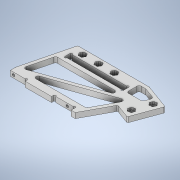
# Autodesk Inventor part: Trunk_vertical_frame_01
Saved by Autodesk Inventor 2020.4 (Build 244396000, 396)
## iProperties
Created: 2021-09-11
Part Number: Trunk_vertical_frame_01
Material: アルミニウム 2014-T4
Document SubType Name: Modeling
Designer: Masato Kubotera
Density: 2.8 g/cm^3
Appearance: 滑らか - 淡い灰色
Mass: 32.437 g
Surface Area: 89.3164 cm^2
Volume: 11.5847 cm^3
Author: Masato Kubotera
Autodesk Inventor part; units mm, degrees
ref_plane "YZ Plane" through (0, 0, 0) normal (1, 0, 0) x (0, 1, 0)
ref_plane "XZ Plane" through (0, 0, 0) normal (0, 1, 0) x (-1, 0, 0)
ref_plane "XY Plane" through (0, 0, 0) normal (0, 0, 1) x (1, 0, 0)
derived "Trunk_vertical_frame_03.ipt"
sketch "スケッチ1" plane through (0, 0, 0) normal (0, 0, 1) x (1, 0, 0)
  circle A0 centre (0, 0) radius 11 projected
  line L0 (1, 13.5) -> (28, 13.5) construction
  line L1 (28, 13.5) -> (28, -13.5) construction
  line L2 (28, -13.5) -> (1, -13.5) construction
  line L3 (1, -13.5) -> (1, 13.5) construction
  line L4 (1, 13.5) -> (28, -13.5) construction
  line L5 (28, 13.5) -> (1, -13.5) construction
  line L6 (-12, 16) -> (39.5, 16) construction
  line L7 (39.5, 16) -> (39.5, -16) construction
  line L8 (39.5, -16) -> (-12, -16) construction
  line L9 (-12, -16) -> (-12, 16) construction
  line L10 (-12, 16) -> (39.5, -16) construction
  line L11 (39.5, 16) -> (-12, -16) construction
  circle A1 centre (1, 13.5) radius 1.35 projected
  arc A2 (0, 16) -> (-12, 10.583) centre (0, 0) ccw construction
  line L12 (-12, 0) -> (39.5, 0) projected
  circle A3 centre (28, 13.5) radius 1.35 projected
  arc A4 (-12, -10.583) -> (0, -16) centre (0, 0) ccw construction
  circle A5 centre (28, -13.5) radius 1.35 projected
  circle A6 centre (1, -13.5) radius 1.35 projected
  arc A7 (0, 16.01) -> (-12.01, 10.5868) centre (0, 0) ccw projected
  line L13 (0, 16.01) -> (39.51, 16.01) projected
  line L14 (39.51, 16.01) -> (39.51, 13.26) projected
  line L15 (-12.01, 10.5868) -> (-12.01, 0) projected
  arc A8 (-11.4729, 11.1666) -> (-12.01, 9.8444) centre (-11.0278, 10.2156) ccw projected
  line L16 (-12.01, 10.5868) -> (-11.0278, 10.2156) construction
  arc A9 (39.51, 14.5251) -> (38.0251, 16.01) centre (38.7675, 15.2675) ccw projected
  line L17 (38.7675, 15.2675) -> (39.51, 16.01) construction
  arc A10 (38.0251, -16.01) -> (39.51, -14.5251) centre (38.7675, -15.2675) ccw projected
  line L18 (-12.01, -10.5868) -> (-12.01, 0) projected
  arc A11 (-12.01, -9.8444) -> (-11.4729, -11.1666) centre (-11.0278, -10.2156) ccw projected
  arc A12 (-12.01, -10.5868) -> (0, -16.01) centre (0, 0) ccw projected
  line L19 (0, -16.01) -> (39.51, -16.01) projected
  line L20 (39.51, 13.26) -> (42.01, 13.26) projected
  line L21 (42.01, 13.26) -> (42.01, -1.76) projected
  line L22 (42.01, -1.76) -> (39.51, -1.76) projected
  line L23 (39.51, -1.76) -> (39.51, -14.5251) projected
  line L24 (39.5, 13.25) -> (42, 13.25) construction
  line L25 (42, 13.25) -> (42, -1.75) construction
  line L26 (42, -1.75) -> (39.5, -1.75) construction
  line L27 (42, 5.75) -> (39.5, 5.75) construction
  arc A13 (42.01, 11.7751) -> (40.5251, 13.26) centre (41.2675, 12.5175) ccw projected
  line L28 (41.2675, 12.5175) -> (42.01, 13.26) construction
  arc A14 (40.5251, -1.76) -> (42.01, -0.2751) centre (41.2675, -1.0175) ccw projected
  circle A15 centre (-15.5, 19) radius 1.55 projected
  line L29 (-18, 22) -> (-13, 22) construction
  line L30 (-13, 22) -> (-13, -10.5) construction
  line L31 (-13, -10.5) -> (-18, -10.5) construction
  line L32 (-18, -10.5) -> (-18, 22) construction
  line L33 (-18, 22) -> (-13, -10.5) construction
  line L34 (-13, 22) -> (-18, -10.5) construction
  line L35 (-18, 5.75) -> (-13, 5.75) construction
  line L36 (-15.5, 22) -> (-15.5, -10.5) construction
  line L37 (-18, 13.25) -> (-15.5, 13.25) construction
  line L38 (-15.5, 13.25) -> (-15.5, -1.75) construction
  line L39 (-15.5, -1.75) -> (-18, -1.75) construction
  line L40 (-18, 13.25) -> (-15.5, -1.75) construction
  line L41 (-15.5, 13.25) -> (-18, -1.75) construction
  line L42 (-15.49, -1.76) -> (-18.01, -1.76) projected
  line L43 (-18.01, -1.76) -> (-18.01, 13.26) projected
  line L44 (-18.01, 13.26) -> (-15.49, 13.26) projected
  line L45 (-15.49, 13.26) -> (-15.49, -1.76) projected
  line L46 (-15.49, -1.76) -> (-18.01, 13.26) construction
  line L47 (-18.01, -1.76) -> (-15.49, 13.26) construction
  line L48 (-16.75, 13.26) -> (-16.75, -1.76) construction
  arc A16 (-18.01, 13.26) -> (-18.01, 11.16) centre (-18.01, 12.21) ccw projected
  arc A17 (-15.49, 11.16) -> (-15.49, 13.26) centre (-15.49, 12.21) ccw projected
  arc A18 (-18.01, 0.34) -> (-18.01, -1.76) centre (-18.01, -0.71) ccw projected
  arc A19 (-15.49, -1.76) -> (-15.49, 0.34) centre (-15.49, -0.71) ccw projected
  circle A20 centre (-15.5, -7.5) radius 1.55 projected
  line L49 (14.5, 16) -> (14.5, -16) construction
  circle A21 centre (42, 19) radius 1.55 projected
  line L50 (39.5, 22) -> (44.5, 22) construction
  line L51 (44.5, 22) -> (44.5, -10.5) construction
  line L52 (44.5, -10.5) -> (39.5, -10.5) construction
  line L53 (39.5, 22) -> (44.5, -10.5) construction
  line L54 (44.5, 22) -> (39.5, -10.5) construction
  line L55 (42, 22) -> (42, -10.5) construction
  circle A22 centre (42, -7.5) radius 1.55 projected
  line L56 (-12, -18.25) -> (27, -18.25) construction
  line L57 (27, -18.25) -> (27, -23.25) construction
  line L58 (27, -23.25) -> (-12, -23.25) construction
  line L59 (-12, -23.25) -> (-12, -18.25) construction
  line L60 (-12, -18.25) -> (27, -23.25) construction
  line L61 (27, -18.25) -> (-12, -23.25) construction
  line L62 (-3, -20.75) -> (18, -20.75) construction
  line L63 (18, -20.75) -> (18, -18.25) construction
  line L64 (-3, -18.25) -> (-3, -20.75) construction
  line L65 (-3, -20.75) -> (18, -18.25) construction
  line L66 (18, -20.75) -> (-3, -18.25) construction
  line L67 (-12, -20.75) -> (27, -20.75) construction
  line L68 (7.5, -18.25) -> (7.5, -23.25) construction
  line L69 (-3.01, -18.24) -> (18.01, -18.24) projected
  line L70 (18.01, -18.24) -> (18.01, -20.76) projected
  line L71 (18.01, -20.76) -> (-3.01, -20.76) projected
  line L72 (-3.01, -20.76) -> (-3.01, -18.24) projected
  line L73 (-3.01, -18.24) -> (18.01, -20.76) construction
  line L74 (18.01, -18.24) -> (-3.01, -20.76) construction
  circle A23 centre (-8, -20.75) radius 1.55 projected
  circle A24 centre (23, -20.75) radius 1.55 projected
  arc A25 (-0.91, -18.24) -> (-3.01, -18.24) centre (-1.96, -18.24) ccw projected
  arc A26 (18.01, -18.24) -> (15.91, -18.24) centre (16.96, -18.24) ccw projected
  line L75 (-3.01, -19.5) -> (18.01, -19.5) construction
  arc A27 (-3.01, -20.76) -> (-0.91, -20.76) centre (-1.96, -20.76) ccw projected
  arc A28 (15.91, -20.76) -> (18.01, -20.76) centre (16.96, -20.76) ccw projected
  circle A29 centre (-8, 20.75) radius 1.55 projected
  line L76 (18.01, 20.76) -> (-3.01, 20.76) projected
  line L77 (-3.01, 19.5) -> (18.01, 19.5) construction
  line L78 (-3, 18.25) -> (-3, 20.75) construction
  line L79 (18, 20.75) -> (-3, 18.25) construction
  line L80 (-3, 20.75) -> (18, 18.25) construction
  line L81 (-3.01, 20.76) -> (-3.01, 18.24) projected
  line L82 (-3.01, 18.24) -> (18.01, 20.76) construction
  line L83 (-3.01, 18.24) -> (18.01, 18.24) projected
  arc A30 (-3.01, 18.24) -> (-0.91, 18.24) centre (-1.96, 18.24) ccw projected
  line L84 (18.01, 18.24) -> (-3.01, 20.76) construction
  line L85 (-12, 23.25) -> (-12, 18.25) construction
  arc A31 (-0.91, 20.76) -> (-3.01, 20.76) centre (-1.96, 20.76) ccw projected
  line L86 (7.5, 18.25) -> (7.5, 23.25) construction
  line L87 (-3, 20.75) -> (18, 20.75) construction
  line L88 (-12, 20.75) -> (27, 20.75) construction
  line L89 (27, 23.25) -> (-12, 23.25) construction
  line L90 (-12, 18.25) -> (27, 18.25) construction
  line L91 (-12, 18.25) -> (27, 23.25) construction
  line L92 (27, 18.25) -> (-12, 23.25) construction
  line L93 (27, 18.25) -> (27, 23.25) construction
  arc A32 (15.91, 18.24) -> (18.01, 18.24) centre (16.96, 18.24) ccw projected
  circle A33 centre (23, 20.75) radius 1.55 projected
  line L94 (18, 20.75) -> (18, 18.25) construction
  line L95 (18.01, 18.24) -> (18.01, 20.76) projected
  arc A34 (18.01, 20.76) -> (15.91, 20.76) centre (16.96, 20.76) ccw projected
  line L96 (-18, 28.25) -> (44.5, 28.25) projected
  line L97 (-18, 28.25) -> (-23, 22) projected
  line L98 (44.5, 28.25) -> (47.5, 22) projected
  line L99 (-23, 22) -> (-23, -2.875) projected
  line L100 (47.5, 22) -> (47.5, -18.25) projected
  line L101 (47.5, -18.25) -> (37, -33.25) projected
  line L102 (-23, -2.875) -> (-33.5, -16) projected
  line L103 (-33.5, -16) -> (-33.5, -87) projected
  line L104 (37, -33.25) -> (37, -73.9) projected
  line L105 (37, -73.9) -> (23, -97) construction
  line L106 (23, -97) -> (-17, -97) construction
  line L107 (-17, -97) -> (-33.5, -87) construction
  circle A35 centre (-12, -92) radius 1.55 projected
  circle A36 centre (3, -92) radius 1.55 projected
  line L108 (-17, -97) -> (-17, -87) construction
  line L109 (-17, -87) -> (23, -87) construction
  line L110 (23, -87) -> (23, -97) construction
  line L111 (-17, -92) -> (23, -92) construction
  line L112 (3, -87) -> (3, -97) construction
  circle A37 centre (18, -92) radius 1.55 projected
  circle A38 centre (-13.5, -58.25) radius 1.55 projected
  line L113 (-23.5, -62.25) -> (27, -62.25) projected
  line L114 (27, -62.25) -> (27, -77) projected
  line L115 (27, -77) -> (-23.5, -77) projected
  line L116 (-23.5, -77) -> (-23.5, -62.25) projected
  line L117 (-23.5, -33.25) -> (27, -33.25) projected
  line L118 (27, -33.25) -> (27, -54.25) projected
  line L119 (27, -54.25) -> (-23.5, -54.25) projected
  line L120 (-23.5, -54.25) -> (-23.5, -33.25) projected
  circle A39 centre (-13.5, -58.25) radius 4 construction
  arc A40 (-11.4565, -94.76) -> (-9.8815, -93.8507) centre (-10.9315, -93.8507) ccw projected
  line L121 (-9.338, -92.9093) -> (-9.8815, -93.8507) projected
  arc A41 (-9.338, -92.9093) -> (-9.338, -91.0907) centre (-9.863, -92) ccw projected
  line L122 (-9.8815, -90.1493) -> (-9.338, -91.0907) projected
  arc A42 (-9.8815, -90.1493) -> (-11.4565, -89.24) centre (-10.9315, -90.1493) ccw projected
  line L123 (-12.5435, -89.24) -> (-11.4565, -89.24) projected
  arc A43 (-12.5435, -89.24) -> (-14.1185, -90.1493) centre (-13.0685, -90.1493) ccw projected
  line L124 (-14.662, -91.0907) -> (-14.1185, -90.1493) projected
  arc A44 (-14.662, -91.0907) -> (-14.662, -92.9093) centre (-14.137, -92) ccw projected
  line L125 (-14.1185, -93.8507) -> (-14.662, -92.9093) projected
  arc A45 (-14.1185, -93.8507) -> (-12.5435, -94.76) centre (-13.0685, -93.8507) ccw projected
  line L126 (-11.4565, -94.76) -> (-12.5435, -94.76) projected
  arc A46 (5.662, -92.9093) -> (5.662, -91.0907) centre (5.137, -92) ccw projected
  line L127 (5.1185, -90.1493) -> (5.662, -91.0907) projected
  line L128 (5.662, -92.9093) -> (5.1185, -93.8507) projected
  arc A47 (3.5435, -94.76) -> (5.1185, -93.8507) centre (4.0685, -93.8507) ccw projected
  arc A48 (5.1185, -90.1493) -> (3.5435, -89.24) centre (4.0685, -90.1493) ccw projected
  line L129 (2.4565, -89.24) -> (3.5435, -89.24) projected
  arc A49 (2.4565, -89.24) -> (0.8815, -90.1493) centre (1.9315, -90.1493) ccw projected
  line L130 (0.338, -91.0907) -> (0.8815, -90.1493) projected
  arc A50 (0.338, -91.0907) -> (0.338, -92.9093) centre (0.863, -92) ccw projected
  line L131 (0.8815, -93.8507) -> (0.338, -92.9093) projected
  arc A51 (0.8815, -93.8507) -> (2.4565, -94.76) centre (1.9315, -93.8507) ccw projected
  line L132 (3.5435, -94.76) -> (2.4565, -94.76) projected
  arc A52 (20.662, -92.9093) -> (20.662, -91.0907) centre (20.137, -92) ccw projected
  line L133 (20.1185, -90.1493) -> (20.662, -91.0907) projected
  line L134 (20.662, -92.9093) -> (20.1185, -93.8507) projected
  arc A53 (18.5435, -94.76) -> (20.1185, -93.8507) centre (19.0685, -93.8507) ccw projected
  arc A54 (20.1185, -90.1493) -> (18.5435, -89.24) centre (19.0685, -90.1493) ccw projected
  line L135 (17.4565, -89.24) -> (18.5435, -89.24) projected
  arc A55 (17.4565, -89.24) -> (15.8815, -90.1493) centre (16.9315, -90.1493) ccw projected
  line L136 (15.338, -91.0907) -> (15.8815, -90.1493) projected
  arc A56 (15.338, -91.0907) -> (15.338, -92.9093) centre (15.863, -92) ccw projected
  line L137 (15.8815, -93.8507) -> (15.338, -92.9093) projected
  arc A57 (15.8815, -93.8507) -> (17.4565, -94.76) centre (16.9315, -93.8507) ccw projected
  line L138 (18.5435, -94.76) -> (17.4565, -94.76) projected
  line L139 (-33.5, -87) -> (46, -87)
  line L140 (46, -87) -> (46, -116.797) construction
  line L141 (46, -116.797) -> (33, -141)
  line L142 (-33.5, -87) -> (-33.5, -139)
  line L143 (-33.5, -139) -> (28.01, -139)
  arc A58 (-17.5, -139) -> (-19.6, -139) centre (-18.55, -139) ccw
  line L144 (-17.5, -139) -> (-17.5, -141)
  line L145 (7.5, -141) -> (7.5, -139)
  arc A59 (9.6, -139) -> (7.5, -139) centre (8.55, -139) ccw
  line L146 (-30.5, -139) -> (-30.5, -141) construction
  line L147 (-33.5, -139) -> (-33.5, -141) construction
  line L148 (28, -139) -> (28, -141) construction
  line L149 (25, -139) -> (25, -141) construction
  line L150 (-33.5, -141) -> (7.5, -141) construction
  line L151 (7.5, -141) -> (33, -141) construction
  line L152 (28.01, -139) -> (34.0742, -139) construction
  arc A60 (28.01, -139) -> (25.91, -139) centre (26.96, -139) ccw
  line L153 (-19, -97) -> (36.5, -97) construction
  line L154 (36.5, -97) -> (36.5, -102) construction
  line L155 (36.5, -102) -> (-19, -102) construction
  line L156 (-19, -102) -> (-19, -97) construction
  line L157 (-19, -99.5) -> (36.5, -99.5) construction
  line L158 (8.75, -97) -> (8.75, -102) construction
  line L159 (-19.05, -96.95) -> (36.55, -96.95)
  line L160 (36.55, -96.95) -> (36.55, -102.05)
  line L161 (36.55, -102.05) -> (-19.05, -102.05)
  line L162 (-19.05, -102.05) -> (-19.05, -96.95)
  line L163 (-19.05, -96.95) -> (36.55, -102.05) construction
  line L164 (36.55, -96.95) -> (-19.05, -102.05) construction
  arc A61 (-16.95, -96.95) -> (-19.05, -96.95) centre (-18, -96.95) ccw
  arc A62 (36.55, -96.95) -> (34.45, -96.95) centre (35.5, -96.95) ccw
  arc A63 (-19.05, -102.05) -> (-16.95, -102.05) centre (-18, -102.05) ccw
  arc A64 (34.45, -102.05) -> (36.55, -102.05) centre (35.5, -102.05) ccw
  line L165 (46, -87) -> (69.5821, -95.5832)
  line L166 (69.5821, -95.5832) -> (60.0056, -121.8946)
  line L167 (60.0056, -121.8946) -> (46, -116.797)
  line L168 (46, -101.8985) -> (64.7939, -108.7389) construction
  circle A65 centre (61.8919, -99.1692) radius 6 construction
  line L169 (61.8919, -99.1692) -> (59.1557, -106.6868) construction
  circle A66 centre (61.8919, -99.1692) radius 2.25
  line L170 (60.8018, -102.164) -> (58.7533, -99.7226)
  line L171 (58.7533, -99.7226) -> (59.8433, -96.7279)
  line L172 (59.8433, -96.7279) -> (62.9819, -96.1745)
  line L173 (62.9819, -96.1745) -> (65.0304, -98.6158)
  line L174 (65.0304, -98.6158) -> (63.9404, -101.6106)
  line L175 (63.9404, -101.6106) -> (60.8018, -102.164)
  arc A67 (60.1269, -101.3597) -> (61.8359, -101.9817) centre (61.161, -101.1773) ccw
  arc A68 (62.9064, -101.7929) -> (64.2995, -100.6239) centre (63.2655, -100.8062) ccw
  arc A69 (64.6713, -99.6025) -> (64.3555, -97.8115) centre (63.9964, -98.7981) ccw
  arc A70 (63.6568, -96.9788) -> (61.9478, -96.3568) centre (62.6227, -97.1611) ccw
  arc A71 (60.8774, -96.5455) -> (59.4842, -97.7145) centre (60.5182, -97.5322) ccw
  arc A72 (59.1124, -98.736) -> (59.4282, -100.527) centre (59.7873, -99.5403) ccw
  circle A73 centre (56.4195, -114.2043) radius 2.25
  line L176 (57.5095, -111.2095) -> (54.371, -111.7629)
  line L177 (54.371, -111.7629) -> (53.281, -114.7577)
  line L178 (53.281, -114.7577) -> (55.3295, -117.1991)
  line L179 (55.3295, -117.1991) -> (58.4681, -116.6457)
  line L180 (58.4681, -116.6457) -> (59.5581, -113.6509)
  line L181 (59.5581, -113.6509) -> (57.5095, -111.2095)
  arc A74 (58.1845, -112.0139) -> (56.4755, -111.3919) centre (57.1504, -112.1962) ccw
  arc A75 (59.199, -114.6376) -> (58.8832, -112.8466) centre (58.524, -113.8332) ccw
  arc A76 (57.434, -116.828) -> (58.8272, -115.659) centre (57.7932, -115.8413) ccw
  arc A77 (54.6546, -116.3947) -> (56.3636, -117.0168) centre (55.6886, -116.2124) ccw
  arc A78 (53.6401, -113.771) -> (53.9559, -115.5621) centre (54.315, -114.5754) ccw
  arc A79 (55.405, -111.5806) -> (54.0119, -112.7496) centre (55.0459, -112.5673) ccw
  line L182 (47.3372, -107.9674) -> (33.3545, -134)
  line L183 (33.3545, -134) -> (-25.927, -134)
  line L184 (-25.927, -134) -> (47.3372, -107.9674)
  line L185 (-29.9686, -132.2523) -> (43.9139, -106)
  line L186 (43.9139, -106) -> (-23.3824, -106)
  line L187 (-23.3824, -106) -> (-29.9686, -132.2523)
  line L188 (-21.7087, -87) -> (-33.5, -134)
  line L189 (-30.407, -134) -> (48.3939, -106) construction
  line L190 (-25.927, -134) -> (-33.5, -134) construction
  line L191 (28.01, -143) -> (31.9258, -143)
  line L192 (28.01, -139) -> (28.01, -143)
  line L193 (33, -141) -> (31.9258, -143)
  circle A80 centre (56.4195, -114.2043) radius 6 construction
  line L194 (39.5, -102) -> (39.5, -90.1925)
  line L195 (39.5, -90.1925) -> (46, -90.1925)
  line L196 (46, -90.1925) -> (57.2798, -94.298)
  line L197 (57.2798, -94.298) -> (54.4765, -102)
  line L198 (54.4765, -102) -> (39.5, -102)
  circle A81 centre (61.8919, -99.1692) radius 1.55
  circle A82 centre (56.4195, -114.2043) radius 1.55
  line L199 (-17.5, -141) -> (7.5, -141)
  point P0 (14.5, 0)
  point P1 (-15.5, 5.75)
  point P2 (-16.75, 5.75)
  point P3 (14.5, 0)
  point P4 (42, 5.75)
  point P5 (42, 5.75)
  point P6 (7.5, -20.75)
  point P7 (7.5, -19.5)
  point P8 (7.5, -19.5)
  point P9 (7.5, -19.5)
  point P10 (7.5, -19.5)
  point P11 (7.5, 20.75)
  point P12 (7.5, 19.5)
  point P13 (7.5, 19.5)
  point P14 (7.5, 19.5)
  point P15 (7.5, 19.5)
  point P16 (3, -89.25)
  point P17 (-10.4065, -94.76)
  point P18 (-8.813, -92)
  point P19 (-10.4065, -89.24)
  point P20 (-13.5935, -89.24)
  point P21 (-13.5935, -89.24)
  point P22 (-15.187, -92)
  point P23 (-13.5935, -94.76)
  point P24 (-15.187, -92)
  point P25 (-8.813, -92)
  point P26 (3, -92)
  point P27 (6.187, -92)
  point P28 (6.187, -92)
  point P29 (4.5935, -89.24)
  point P30 (4.5935, -94.76)
  point P31 (3, -92)
  point P32 (3, -92)
  point P33 (1.4065, -89.24)
  point P34 (1.4065, -89.24)
  point P35 (-0.187, -92)
  point P36 (-0.187, -92)
  point P37 (1.4065, -94.76)
  point P38 (18, -92)
  point P39 (21.187, -92)
  point P40 (21.187, -92)
  point P41 (19.5935, -89.24)
  point P42 (19.5935, -94.76)
  point P43 (18, -92)
  point P44 (18, -92)
  point P45 (16.4065, -89.24)
  point P46 (16.4065, -89.24)
  point P47 (14.813, -92)
  point P48 (14.813, -92)
  point P49 (16.4065, -94.76)
  point P50 (3, -87)
  point P51 (8.75, -99.5)
  point P52 (63.9404, -101.6106)
  point P53 (65.0304, -98.6158)
  point P54 (62.9819, -96.1745)
  point P55 (59.8433, -96.7279)
  point P56 (58.7533, -99.7226)
  point P57 (59.5581, -113.6509)
  point P58 (58.4681, -116.6457)
  point P59 (55.3295, -117.1991)
  point P60 (53.281, -114.7577)
  point P61 (54.371, -111.7629)
  point P62 (34.45, -102.05)
  point P63 (-16.95, -102.05)
  point P64 (34.45, -96.95)
  point P65 (-14.1185, -90.1493)
  point P66 (0.8815, -90.1493)
  point P67 (15.8815, -90.1493)
  point P68 (57.434, -116.828)
  point P69 (56.3636, -117.0168)
  point P70 (54.6546, -116.3947)
  point P71 (53.9559, -115.5621)
  point P72 (53.6401, -113.771)
  point P73 (54.0119, -112.7496)
  point P74 (55.405, -111.5806)
  point P75 (58.8832, -112.8466)
  point P76 (59.199, -114.6376)
  point P77 (58.8272, -115.659)
  point P78 (59.1124, -98.736)
  point P79 (59.4842, -97.7145)
  point P80 (60.8774, -96.5455)
  point P81 (61.9478, -96.3568)
  point P82 (63.6568, -96.9788)
  point P83 (64.3555, -97.8115)
  point P84 (64.6713, -99.6025)
  point P85 (64.2995, -100.6239)
  point P86 (62.9064, -101.7929)
  point P87 (59.4282, -100.527)
  point P88 (7.5, -139)
  point P89 (7.5, -139)
  dimension "d2" = 1.05
  dimension "d7" = 1.05
  dimension "d12" = 2
  dimension "d16" = 3
  dimension "d17" = 3
  dimension "d21" = 61.5
  dimension "d22" = 5
  dimension "d23" = 1.05
  dimension "d24" = 42
  dimension "d25" = 43
  dimension "d27" = 0.05
  dimension "d28" = 0.05
  dimension "d29" = 5
  dimension "d30" = 55.5
  dimension "d31" = 1.05
  dimension "d33" = 22
  dimension "d34" = 12
  dimension "d36" = 4.5
  dimension "d37" = 5.52
  dimension "d38" = 1.05
  dimension "d41" = 360
  dimension "d43" = 16
  dimension "d44" = 3
  dimension "d47" = 5
  dimension "d48" = 4
  dimension "d50" = 3
  dimension "d52" = 1.5
  dimension "d53" = 1.5
  dimension "d55" = 5
  dimension "d73" = 5
  dimension "d74" = 4
  dimension "d75" = 0.01
  dimension "d76" = 110
  dimension "d77" = 20
  dimension "d78" = 3
  dimension "d79" = 3
  dimension "d80" = 3.1
  dimension "d83" = 25
  dimension "d84" = 16
  constraints: 121 end point, 40 symmetric about line, 39 point on circle, 25 centre point, 23 point on line, 19 perpendicular, 10 midpoint, 9 horizontal, 9 parallel, 6 tangent, 5 coincident, 5 collinear, 4 vertical, 71 other
  measures "d2" radius of A58
  measures "d7" radius of A59
  measures "d12" distance of L142.end L147.end
  measures "d16" distance of L147.end L146.end
  measures "d17" distance of L148.end L149.end
  measures "d21" distance of L147.end L148.end
  measures "d22" distance of L141.end L148.end
  measures "d23" radius of A60
  measures "d24" vertical distance of L142.end L106.end
  measures "d25" distance of L139.end L112.start
  measures "d27" horizontal distance of L159.start L153.start
  measures "d28" horizontal distance of L153.start L159.start
  measures "d29" distance of L155.end L153.start
  measures "d30" distance of L157.end L157.start
  measures "d31" radius of A61
  measures "d33" horizontal distance of L153.start point (3, -92)
  measures "d34" diameter of A65
  measures "d36" diameter of A66
  measures "d37" distance from line of L172 L174.end
  measures "d38" radius of A67
  measures "d43" distance of point (56.42, -114.204) A66.centre
  measures "d44" distance between parallel lines of L141 L182
  measures "d47" distance of L188.end L142.end
  measures "d48" vertical distance of L186.end L155.end
  measures "d50" distance between parallel lines of L188 L187
  measures "d52" distance between parallel lines of L184 L189
  measures "d53" distance between parallel lines of L189 L185
  measures "d55" distance from line of L159.start L188
  measures "d73" vertical distance of A35.centre L153.start
  measures "d74" distance between parallel lines of L191 L152
  measures "d75" distance between parallel lines of L192 L148
  measures "d76" angle of L140 L168
  measures "d77" distance of L168.start L168.end
  measures "d78" distance between parallel lines of L196 L165
  measures "d79" distance between parallel lines of L154 L194
  measures "d80" diameter of A81
  measures "d83" distance of L145.start L144.end
  measures "d84" horizontal distance of L144.end L142.end
extrude "押し出し1" add sketch "スケッチ1" along normal blind 5 contours L139 L165 L166 L167 L141 L193 L191 L192 A60 L143 A59 A58 L142 L188 | L143 L145 L199 L144
sketch "スケッチ2" plane through (-33.5, -139, 0) normal (0, -1, 0) x (1, 0, 0)
  line L0 (41, 0) -> (41, 5) projected
  line L1 (61.51, 0) -> (61.51, 5) projected
  line L2 (16, 0) -> (16, 5) projected
  point P0 (33.5, 0)
  point P1 (3, 2.5)
  point P2 (0, 0)
  point P3 (54, 2.5)
  dimension "d59" = 2.5
  dimension "d61" = 2.5
  dimension "d86" = 13
  dimension "d87" = 13
  measures "d59" vertical distance of point (0, 0) point (3, 2.5)
  measures "d61" vertical distance of point (0, 0) point (54, 2.5)
  measures "d86" distance from line of point (3, 2.5) L2
  measures "d87" distance from line of point (54, 2.5) L0
hole "穴1" at (-30.5, -139, 2.5) at (20.5, -139, 2.5) direction (0, 1, 0) diameter 2.459 depth 5 thread size "M3x0.5" class "6H" standard "ISO Metric profile"
fillet "フィレット1" radius 1 6 edges at (-21.7087, -87, 2.5) (69.5821, -95.5832, 2.5) (60.0056, -121.8946, 2.5) (46, -116.797, 2.5) (46, -87, 2.5) (-33.5, -134, 2.5)
extrude "押し出し2" add sketch "スケッチ1" along normal blind 2.8 contours A67 L170 | L170 L171 L172 L173 L174 L175 | L175 A67 | A72 L170 | L175 A68 | A72 L171 | L174 A68 | A71 L171 | L174 A69 | A71 L172 | L173 A69 | A70 L172 | L173 A70 | L181 L180 L179 L178 L177 L176 | A74 L181 | L176 A74 | L176 A79 | A75 L181 | L177 A79 | A75 L180 | L177 A78 | A76 L180 | L178 A78 | A76 L179 | L178 A77 | A77 L179
fillet "フィレット2" radius 2 10 edges at (-23.3824, -106, 2.5) (-29.9686, -132.2523, 2.5) (-25.927, -134, 2.5) (43.9139, -106, 2.5) (33.3545, -134, 2.5) (47.3372, -107.9674, 2.5) (39.5, -90.1925, 2.5) (39.5, -102, 2.5) (54.4765, -102, 2.5) (57.2798, -94.298, 2.5)
extrude "押し出し3" add sketch "スケッチ1" along normal blind 2 contours A66 | A73
equation "\"d7\" = d2"
equation "\"d23\" = d7"
equation "\"d28\" = d27"
equation "\"d31\" = d2"
equation "\"d38\" = d2"
equation "\"d50\" = d49"
equation "\"d13\" = d10"
equation "\"d49\" = 3"
equation "\"d10\" = 0.01"
